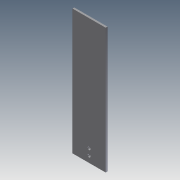
# Autodesk Inventor part: back
Saved by Autodesk Inventor 2011 (Build 150239000, 239)
## iProperties
Created: 2011-10-08
Part Number: back
Document SubType Name: Modeling
Designer: Matthew
Density: 1 g/cm^3
Author: Matthew
Autodesk Inventor part; units mm, degrees
ref_plane "YZ Plane" through (0, 0, 0) normal (1, 0, 0) x (0, 1, 0)
ref_plane "XZ Plane" through (0, 0, 0) normal (0, 1, 0) x (-1, 0, 0)
ref_plane "XY Plane" through (0, 0, 0) normal (0, 0, 1) x (1, 0, 0)
sketch "Sketch1" plane through (0, 0, 0) normal (0, 0, 1) x (1, 0, 0)
  line L0 (-22.2985, 25.8576) -> (117.4015, 25.8576)
  line L1 (117.4015, 25.8576) -> (117.4015, -278.9424)
  line L2 (117.4015, -278.9424) -> (-22.2985, -278.9424)
  line L3 (-22.2985, -278.9424) -> (-22.2985, 25.8576)
  point P0 (0, 0)
  dimension "d0" = 139.7
  dimension "d1" = 304.8
  constraints: 8 end point, 2 parallel, 1 horizontal, 1 perpendicular
  measures "d0" distance of L1.end L2.end
  measures "d1" distance of L0.end L1.end
extrude "Extrusion1" add sketch "Sketch1" along normal blind 6.35
sketch "Sketch2" plane through (117.4015, -278.9424, 0) normal (1, 0, 0) x (0, 0, -1)
  line L0 (-6.35, 304.8) -> (-6.35, 0) projected
  line L1 (0, 0) -> (-6.35, 0) projected
  line L2 (0, 304.8) -> (0, 0) projected
  line L3 (0, 304.8) -> (-6.35, 304.8) projected
  point P0 (0, 278.9424)
extrude "Extrusion2" add sketch "Sketch2" along normal blind 12.7
sketch "Sketch3" plane through (130.1015, -278.9424, 0) normal (1, 0, 0) x (0, 0, -1)
  line L0 (-6.35, 304.8) -> (0, 304.8) projected
  line L1 (-6.35, 0) -> (-6.35, 304.8) projected
  line L2 (0, 0) -> (-6.35, 0) projected
  line L3 (0, 304.8) -> (0, 0) projected
  point P0 (0, 278.9424)
extrude "Extrusion3" cut sketch "Sketch3" against normal blind 38.1
sketch "Sketch5" plane through (0, 0, 6.35) normal (0, 0, 1) x (1, 0, 0)
  line L0 (-22.2985, -278.9424) -> (92.0015, -278.9424)
  line L1 (92.0015, -278.9424) -> (92.0015, -532.9424)
  line L2 (92.0015, -532.9424) -> (-22.2985, -532.9424)
  line L3 (-22.2985, -532.9424) -> (-22.2985, -278.9424)
  point P0 (0, 0)
  dimension "d9" = 254
  constraints: 8 end point, 2 parallel, 1 horizontal, 1 perpendicular
  measures "d9" distance of L0.end L1.end
extrude "Extrusion4" add sketch "Sketch5" against normal blind 6.35
sketch "Sketch6" plane through (-22.2985, -532.9424, 6.35) normal (0, -1, 0) x (1, 0, 0)
  line L0 (0, -6.35) -> (114.3, -6.35) projected
  line L1 (114.3, 0) -> (114.3, -6.35) projected
  line L2 (0, 0) -> (114.3, 0) projected
  line L3 (0, 0) -> (0, -6.35) projected
  point P0 (22.2985, -6.35)
extrude "Extrusion5" cut sketch "Sketch6" against normal blind 127
sketch "Sketch7" plane through (0, 0, 6.35) normal (0, 0, 1) x (1, 0, 0)
  line L0 (-22.2985, -405.9424) -> (92.0015, -405.9424) projected
  line L1 (92.0015, -405.9424) -> (92.0015, 25.8576) projected
  line L2 (-22.2985, -405.9424) -> (92.0015, -405.9424)
  line L3 (92.0015, -405.9424) -> (92.0015, -399.5924)
  line L4 (92.0015, -399.5924) -> (-22.2985, -399.5924)
  line L5 (-22.2985, -399.5924) -> (-22.2985, -405.9424)
  point P0 (0, 0)
  dimension "d14" = 6.35
  constraints: 8 end point, 2 parallel, 1 horizontal, 1 perpendicular, 1 point on line
  measures "d14" distance of L3.end L2.end
extrude "Extrusion6" cut sketch "Sketch7" against normal blind 25.4
sketch "Sketch8" plane through (0, 0, 6.35) normal (0, 0, 1) x (1, 0, 0)
  line L0 (-22.2985, -399.5924) -> (92.0015, -399.5924)
  line L1 (92.0015, -399.5924) -> (92.0015, -405.9424)
  line L2 (92.0015, -405.9424) -> (-22.2985, -405.9424)
  line L3 (-22.2985, -405.9424) -> (-22.2985, -399.5924)
  point P0 (0, 0)
  dimension "d17" = 6.35
  constraints: 8 end point, 2 parallel, 1 horizontal, 1 perpendicular
  measures "d17" distance of L0.end L1.end
extrude "Extrusion7" add sketch "Sketch8" against normal blind 6.35
sketch "Sketch9" plane through (0, 0, 6.35) normal (0, 0, 1) x (1, 0, 0)
  line L0 (-22.2985, -405.9424) -> (92.0015, -405.9424) projected
  line L1 (34.8515, -405.9424) -> (34.8515, -392.6074)
  line L2 (34.8515, -392.6074) -> (34.8515, -384.6074)
  circle A0 centre (34.8515, -384.6074) radius 5
  line L3 (34.8515, -392.6074) -> (34.8515, -362.6074)
  circle A1 centre (34.8515, -362.6074) radius 5
  point P0 (0, 0)
  dimension "d20" = 13.335
  dimension "d21" = 8
  dimension "d22" = 10
  dimension "d23" = 30
  dimension "d24" = 10
  constraints: 6 end point, 2 centre point, 2 coincident, 1 collinear, 1 midpoint, 1 perpendicular, 1 point on line
  measures "d20" distance of L1.start L1.end
  measures "d21" distance of L1.end L2.end
  measures "d22" diameter of A0
  measures "d23" distance of L1.end L3.end
  measures "d24" diameter of A1
extrude "Extrusion8" cut sketch "Sketch9" against normal blind 25.4
sketch "Sketch10" plane through (-22.2985, 25.8576, 6.35) normal (0, 1, 0) x (1, 0, 0)
  line L0 (114.3, 0) -> (114.3, 6.35) projected
  line L1 (0, 6.35) -> (114.3, 6.35) projected
  line L2 (0, 6.35) -> (0, 0) projected
  line L3 (0, 0) -> (114.3, 0) projected
  point P0 (22.2985, 6.35)
extrude "Extrusion9" cut sketch "Sketch10" against normal blind 12.7
sketch "Sketch11" plane through (-22.2985, -405.9424, 6.35) normal (0, -1, 0) x (1, 0, 0)
  line L0 (0, -6.35) -> (114.3, -6.35) projected
  line L1 (114.3, 0) -> (114.3, -6.35) projected
  line L2 (0, 0) -> (114.3, 0) projected
  line L3 (0, 0) -> (0, -6.35) projected
  point P0 (22.2985, -6.35)
extrude "Extrusion10" cut sketch "Sketch11" against normal blind 12.7
body "Solid1"
